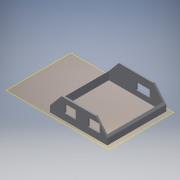
# Autodesk Inventor part: Aussenwände_oben
Saved by Autodesk Inventor 2017 (Build 210142000, 142)
## iProperties
Created: 2017-06-01
Part Number: Aussenwände_oben
Material: Generic
Document SubType Name: Modeling
Designer: Fake
Density: 1 g/cm^3
Appearance: Default
Author: Fake
Autodesk Inventor part; units mm, degrees
ref_plane "YZ Plane" through (0, 0, 0) normal (1, 0, 0) x (0, 1, 0)
ref_plane "XZ Plane" through (0, 0, 0) normal (0, 1, 0) x (-1, 0, 0)
ref_plane "XY Plane" through (0, 0, 0) normal (0, 0, 1) x (1, 0, 0)
ref_plane "Arbeitsebene1" through (0, 0, 3900) normal (0, 0, 1) x (1, 0, 0)
sketch "Skizze1" plane through (0, 0, 3900) normal (0, 0, 1) x (1, 0, 0)
  line L0 (5680, -3575) -> (5680, 3575) projected
  line L1 (5680, 3575) -> (-5680, 3575) projected
  line L2 (-5680, -3575) -> (5680, -3575) projected
  line L3 (-1284.1409, 3575) -> (5680, 3575)
  line L4 (5680, 3575) -> (5680, -3575)
  line L5 (5680, -3575) -> (-1284.1409, -3575)
  line L6 (-1084.1409, 3375) -> (5480, 3375)
  line L7 (5480, 3375) -> (5480, -3375)
  line L8 (5480, -3375) -> (-1084.1409, -3375)
  line L9 (-1284.1409, -3575) -> (-1234.707, -3575)
  line L10 (-1084.1409, -3375) -> (-1084.1409, 3375)
  line L11 (-1234.707, 3575) -> (-1284.1409, 3575)
  line L12 (-1284.1409, 3575) -> (-1284.1409, -3575)
  dimension "d0" = 200
  dimension "d2" = 200
  dimension "d3" = 200
  dimension "d6" = 200
  constraints: 21 end point, 4 parallel, 3 horizontal, 3 perpendicular, 1 collinear, 1 point on line
  measures "d0" distance between parallel lines of L1 L6
  measures "d2" distance between parallel lines of L0 L7
  measures "d3" distance between parallel lines of L8 L2
  measures "d6" distance between parallel lines of L12 L10
extrude "Extrusion1" add sketch "Skizze1" along normal blind 2500
sketch "Skizze2" plane through (-1284.1409, -3575, 3900) normal (0, -1, 0) x (1, 0, 0)
  line L0 (0, 0) -> (6964.1409, 0) projected
  line L1 (6964.1409, 0) -> (6964.1409, 2500) projected
  line L2 (0, 2500) -> (6964.1409, 2500) projected
  line L3 (0, 0) -> (0, 2500) projected
  line L4 (0, 0) -> (0, 2500) projected
  line L5 (0, 728.5709) -> (1486.4055, 2500)
  line L6 (6764.1409, 2500) -> (200, 2500) projected
  line L7 (1486.4055, 2500) -> (0, 2500)
  line L8 (0, 728.5709) -> (0, 2500)
  line L9 (5477.7354, 2500) -> (6964.1409, 728.5709)
  line L10 (6964.1409, 0) -> (6964.1409, 2500) projected
  line L11 (6964.1409, 2500) -> (6964.1409, 728.5709)
  line L12 (6964.1409, 2500) -> (5477.7354, 2500)
  dimension "d13" = 40
  dimension "d14" = 40
  constraints: 12 end point, 4 point on line, 3 collinear, 1 horizontal alignment, 1 vertical
  measures "d13" angle of L5 L3
  measures "d14" angle of L9 L1
extrude "Extrusion2" cut sketch "Skizze2" against normal up to surface (7150 mm away) contours L3 L2 L5 | L9 L2 L1
sketch "Skizze3" plane through (-1284.1409, -3575, 3900) normal (0, -1, 0) x (1, 0, 0)
  line L0 (1486.4055, 2500) -> (0, 728.5709) projected
  line L1 (0, 0) -> (0, 728.5709) projected
  line L2 (0, 0) -> (6964.1409, 0) projected
  line L3 (6964.1409, 0) -> (6964.1409, 728.5709) projected
  line L4 (1486.4055, 2500) -> (5477.7354, 2500) projected
  line L5 (1990.078, 2180) -> (3070.078, 2180)
  line L6 (3070.078, 2180) -> (3070.078, 1000)
  line L7 (3070.078, 1000) -> (1990.078, 1000)
  line L8 (1990.078, 1000) -> (1990.078, 2180)
  line L9 (4244.6225, 2180) -> (5324.6225, 2180)
  line L10 (5324.6225, 2180) -> (5324.6225, 1000)
  line L11 (5324.6225, 1000) -> (4244.6225, 1000)
  line L12 (4244.6225, 1000) -> (4244.6225, 2180)
  line L13 (6964.1409, 728.5709) -> (5477.7354, 2500) projected
  dimension "d15" = 1080
  dimension "d16" = 1080
  dimension "d17" = 1180
  dimension "d18" = 1000
  constraints: 16 end point, 4 parallel, 2 horizontal, 2 perpendicular, 2 point on line
  measures "d15" distance of L5.start L5.end
  measures "d16" distance between parallel lines of L10 L12
  measures "d17" distance of L5.end L6.end
  measures "d18" distance between parallel lines of L7 L2
extrude "Extrusion3" cut sketch "Skizze3" against normal up to surface (200 mm away) contours L5 L6 L7 L8 | L9 L10 L11 L12
sketch "Skizze4" plane through (-1284.1409, 3575, 3900) normal (0, 1, 0) x (1, 0, 0)
  line L0 (5172.9172, -1486.059) -> (3509.2696, -1486.059)
  line L1 (3509.2696, -1486.059) -> (3509.2696, -633.4396)
  line L2 (3509.2696, -633.4396) -> (5172.9172, -633.4396)
  line L3 (5172.9172, -633.4396) -> (5172.9172, -1486.059)
  constraints: 8 end point, 2 parallel, 1 horizontal, 1 perpendicular
extrude "Extrusion4" cut sketch "Skizze4" against normal up to surface (200 mm away)
equation "\"d14\" = d13"
equation "\"d16\" = d15"
